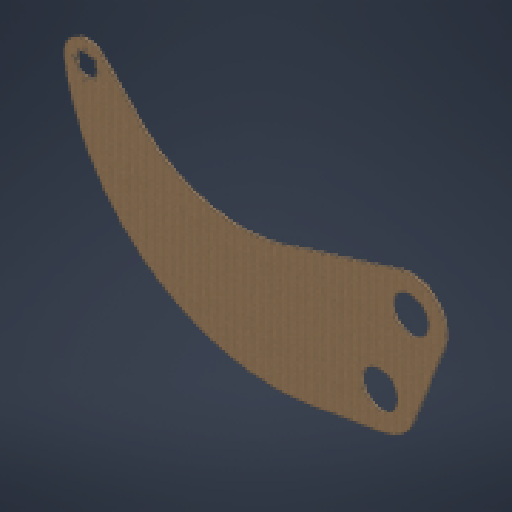
# Autodesk Inventor part: WhipperArm
Saved by Autodesk Inventor 2024.1 (Build 281209000, 209)
## iProperties
Created: 2023-10-16
Part Number: WhipperArm
Material: MDF Medium Density Fiberboard
Document SubType Name: Modeling
Designer: Brandon
Density: 0.8 g/cm^3
Appearance: Cardboard - Corrugated
Author: Brandon
Autodesk Inventor part; units mm, degrees
ref_plane "YZ Plane" through (0, 0, 0) normal (1, 0, 0) x (0, 1, 0)
ref_plane "XZ Plane" through (0, 0, 0) normal (0, 1, 0) x (-1, 0, 0)
ref_plane "XY Plane" through (0, 0, 0) normal (0, 0, 1) x (1, 0, 0)
sketch "Sketch1" plane through (0, 0, 0) normal (0, 0, 1) x (1, 0, 0)
  line L0 (6.4658, -12.7) -> (12.7, -12.7) projected
  arc A0 (-6.4658, -12.7) -> (6.4658, -12.7) centre (0, 0) ccw projected
  line L1 (-12.7, -12.7) -> (-6.4658, -12.7) projected
  line L2 (-12.7, -6.4658) -> (-12.7, -12.7) projected
  arc A1 (-12.7, 6.4658) -> (-12.7, -6.4658) centre (0, 0) ccw projected
  line L3 (-12.7, 12.7) -> (-12.7, 6.4658) projected
  line L4 (-6.4658, 12.7) -> (-12.7, 12.7) projected
  arc A2 (6.4658, 12.7) -> (-6.4658, 12.7) centre (0, 0) ccw projected
  line L5 (12.7, 12.7) -> (6.4658, 12.7) projected
  line L6 (12.7, 6.4658) -> (12.7, 12.7) projected
  arc A3 (12.7, -6.4658) -> (12.7, 6.4658) centre (0, 0) ccw projected
  line L7 (12.7, -12.7) -> (12.7, -6.4658) projected
  arc A4 (22.4506, 22.4506) -> (11.1037, -29.7451) centre (0, 0) ccw projected
  line L8 (53.8815, -8.9803) -> (157.065, -121.1361)
  line L9 (157.065, -121.1361) -> (447.7579, -29.481)
  line L10 (157.065, -121.1361) -> (461.865, -121.1361) construction
  circle A5 centre (463.0337, -77.9298) radius 50.8
  circle A6 centre (419.3415, -191.752) radius 50.8
  line L11 (463.0337, -77.9298) -> (419.3415, -191.752)
  line L12 (463.0337, -77.9298) -> (584.9537, -77.9298) construction
  arc A7 (-31.41, -4.6344) -> (323.0536, -260.3138) centre (270.1256, 39.8556) ccw
  line L13 (428.1628, -241.7802) -> (323.0536, -260.3138)
  line L14 (428.1628, -241.7802) -> (534.8936, -241.7802) construction
  line L15 (510.4596, -96.1349) -> (466.7674, -209.9571)
  circle A8 centre (0, -19.05) radius 2
  circle A9 centre (19.05, 0) radius 2
  circle A10 centre (-19.05, 0) radius 2
  circle A11 centre (0, 19.05) radius 2
  line L16 (22.4506, 22.4506) -> (53.8815, -8.9803) projected
  line L17 (52.7468, -14.1998) -> (11.1037, -29.7451) projected
  arc A12 (52.7468, -14.1998) -> (53.8815, -8.9803) centre (51.6365, -11.2253) ccw projected
  circle A13 centre (0, -19.05) radius 2.735 projected
  circle A14 centre (-19.05, 0) radius 2.735 projected
  circle A15 centre (0, 19.05) radius 2.735 projected
  circle A16 centre (19.05, 0) radius 2.735 projected
  circle A17 centre (463.0337, -77.9298) radius 25.4
  circle A18 centre (419.3415, -191.752) radius 25.4
  point P0 (50.8347, -14.9136)
  point P1 (54.0605, -9.1748)
  dimension "d0" = 152.4
  dimension "d1" = 304.8
  dimension "d2" = 17.5
  dimension "d3" = 101.6
  dimension "d4" = 101.6
  dimension "d5" = 121.92
  dimension "d6" = 111
  dimension "d7" = 609.6
  dimension "d9" = 170
  dimension "d10" = 4
  dimension "d11" = 4
  dimension "d12" = 4
  dimension "d13" = 4
  dimension "d16" = 50.8
  dimension "d17" = 50.8
  constraints: 16 end point, 9 centre point, 7 point on circle, 6 tangent, 3 equal length, 3 horizontal, 2 coincident
  measures "d0" distance of L8.start L8.end
  measures "d1" distance of L8.end L9.end
  measures "d2" angle of L10 L9
  measures "d3" diameter of A5
  measures "d4" diameter of A6
  measures "d5" distance of L11.start L11.end
  measures "d6" angle of L11 L12
  measures "d7" diameter of A7
  measures "d9" angle of L13 L14
  measures "d10" diameter of A8
  measures "d11" diameter of A9
  measures "d12" diameter of A10
  measures "d13" diameter of A11
  measures "d16" diameter of A17
  measures "d17" diameter of A18
extrude "Extrusion1" add sketch "Sketch1" along normal blind 3.175 contours L16 L8 L9 A5 L11 A6 L13 A7 A4 | A6 | A5 | A6 L11 A5 L15 | A13 | A14 | A15 | A16
fillet "Fillet1" radius 203.2 1 edges at (157.065, -121.1361, 1.5875)
body "Solid1"
